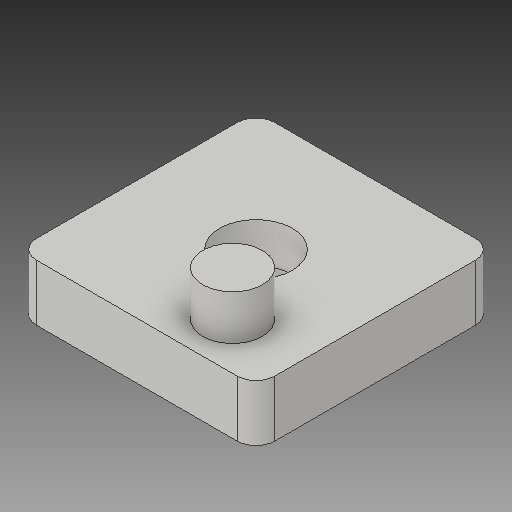
# Autodesk Inventor part: BearingMount
Saved by Autodesk Inventor 2019 (Build 230136000, 136)
## iProperties
Created: 2019-07-17
Part Number: BearingMount
Material: Generic
Document SubType Name: Modeling
Designer: aorfi
Density: 1 g/cm^3
Appearance: Default
Author: aorfi
Autodesk Inventor part; units mm, degrees
ref_plane "YZ Plane" through (0, 0, 0) normal (1, 0, 0) x (0, 1, 0)
ref_plane "XZ Plane" through (0, 0, 0) normal (0, 1, 0) x (-1, 0, 0)
ref_plane "XY Plane" through (0, 0, 0) normal (0, 0, 1) x (1, 0, 0)
sketch "Sketch1" plane through (0, 0, 0) normal (0, 1, 0) x (-1, 0, 0)
  line L0 (-12.7, 12.7) -> (12.7, 12.7)
  line L1 (12.7, 12.7) -> (12.7, -12.7)
  line L2 (12.7, -12.7) -> (-12.7, -12.7)
  line L3 (-12.7, -12.7) -> (-12.7, 12.7)
  line L4 (-12.7, 12.7) -> (12.7, -12.7) construction
  line L5 (12.7, 12.7) -> (-12.7, -12.7) construction
  point P0 (0, 0)
  dimension "d0" = 25.4
  dimension "d1" = 25.4
  constraints: 12 end point, 2 midpoint, 2 parallel, 1 horizontal, 1 perpendicular
  measures "d0" distance of L0.end L1.end
  measures "d1" distance of L1.end L2.end
extrude "Extrusion1" add sketch "Sketch1" along normal mid plane 6
sketch "Sketch2" plane through (0, 3, 0) normal (0, 1, 0) x (1, 0, 0)
  point P0 (0, 0)
hole "Hole1" at (0, 3, 0) direction (0, -1, 0) diameter 4.496 end through all clearance for "Flat Head Machine Screw (82)" size "#8" standard "Ansi Unified Screw Threads"
sketch "Sketch3" plane through (0, 3, 0) normal (0, 1, 0) x (1, 0, 0)
  circle A0 centre (0, 0) radius 3.875
  dimension "d11" = 7.75
  constraints: 1 centre point, 1 coincident
  measures "d11" diameter of A0
extrude "Extrusion2" cut sketch "Sketch3" against normal blind 4.2672
sketch "Sketch4" plane through (0, 3, 0) normal (0, 1, 0) x (1, 0, 0)
  circle A0 centre (5.2, -7.7) radius 3.175
  line L0 (-12.7, -12.7) -> (12.7, -12.7) construction
  line L1 (-2.3, 0) -> (12.7, 0) construction
  line L2 (12.7, -12.7) -> (12.7, 12.7) construction
  point P0 (5.2, 0)
  point P1 (0, 0)
  dimension "d14" = 6.35
  dimension "d17" = 15
  dimension "d18" = 5
  constraints: 2 end point, 2 midpoint, 1 centre point, 1 point on line, 1 vertical alignment
  measures "d14" diameter of A0
  measures "d17" distance of L1.end L1.start
  measures "d18" distance from line of L0 A0.centre
extrude "Extrusion3" add sketch "Sketch4" along normal blind 4.7625
fillet "Fillet1" radius 2 4 edges at (-12.7, 0, 12.7) (12.7, 0, 12.7) (12.7, 0, -12.7) (-12.7, 0, -12.7)
equation "\"d1\" = d0"
body "Solid1"
